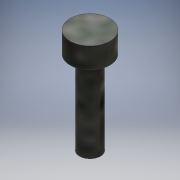
# Autodesk Inventor part: M2 キャップスクリュー　8mm
Saved by Autodesk Inventor 2016 (Build 200138000, 138)
## iProperties
Created: 2017-03-16
Part Number: M2 キャップスクリュー　8mm
Material: 鋼
Document SubType Name: Modeling
Designer: Takumi
Mass: 0.375348 g
Surface Area: 0.968239 cm^2
Volume: 0.047815 cm^3
Density: 7.85 g/cm^3
Appearance: プレート
Author: Takumi
Autodesk Inventor part; units mm, degrees
ref_plane "YZ Plane" through (0, 0, 0) normal (1, 0, 0) x (0, 1, 0)
ref_plane "XZ Plane" through (0, 0, 0) normal (0, 1, 0) x (-1, 0, 0)
ref_plane "XY Plane" through (0, 0, 0) normal (0, 0, 1) x (1, 0, 0)
sketch "スケッチ1" plane through (0, 0, 0) normal (0, 0, 1) x (1, 0, 0)
  circle A0 centre (0, 0) radius 1.9
  circle A1 centre (0, 0) radius 1
  dimension "d0" = 3.8
  dimension "d1" = 2
  constraints: 2 centre point, 2 coincident
  measures "d0" diameter of A0
  measures "d1" diameter of A1
extrude "押し出し1" add sketch "スケッチ1" along normal blind 2 contours A0 | A1
extrude "押し出し2" add sketch "スケッチ1" against normal blind 8 contours A1
